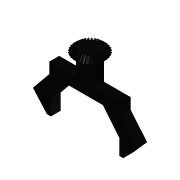
# Autodesk Inventor part: Gripper_Gear
Saved by Autodesk Inventor 2016 (Build 200138000, 138)
## iProperties
Created: 2015-05-21
Part Number: Gripper_Gear
Material: PC/ABS Plastic
Document SubType Name: Modeling
Designer: CHUNGBK
Categories: <?xml version="1.0" encoding="UTF-16"?> <MemberInstance><Categories><FamilyTemplate><FamilyTemplateParameter ValueType="xs:double" Id="1" ObjectReferenceKey="da_z" ObjectType="kUserParameterObject"/><FamilyTemplateParameter ValueType="xs:double" Id="2" ObjectReferenceKey="da_b" ObjectType="kUserParameterObject"/><FamilyTemplateParameter ValueType="xs:double" Id="3" ObjectReferenceKey="da_beta" ObjectType="kUserParameterObject"/><FamilyTemplateParameter ValueType="xs:double" Id="4" ObjectReferenceKey="da_dae" ObjectType="kUserParameterObject"/><FamilyTemplateParameter ValueType="xs:double" Id="5" ObjectReferenceKey="da_ve" ObjectType="kUserParameterObject"/><FamilyTemplateParameter ValueType="xs:double" Id="6" ObjectReferenceKey="da_omega" ObjectType="kUserParameterObject"/><FamilyTemplateParameter ValueType="xs:string" Id="7" ObjectReferenceKey="EAIAABAAAAAAHwAAAAAAAIAAAAAAAAAA" ObjectType="83914240" SubObjectId="SurfaceGeometry"/></FamilyTemplate><ParamToTemplateMap><ParamToTemplate CategoryParameter="//CategoryParameter[@InternalName='046C89C9-8512-4d59-83FE-43B91F4F132A']" TemplateParameter="1"/><ParamToTemplate CategoryParameter="//CategoryParameter[@InternalName='2552DF32-E462-4b46-AEBF-C6C7768E72AC']" TemplateParameter="2"/><ParamToTemplate CategoryParameter="//CategoryParameter[@InternalName='C9EE641D-15FC-4fae-A226-E94C4372FDD7']" TemplateParameter="3"/><ParamToTemplate><ParamToTemplate CategoryParameter="//CategoryParameter[@InternalName='00B6519A-459B-49c7-AD84-2E56D39A5744']" ConstantValue="0.000000"/></ParamToTemplate><ParamToTemplate><ParamToTemplate CategoryParameter="//CategoryParameter[@InternalName='04B31F0E-C7A6-4894-AA32-9629BEFACF47']" ConstantValue="1.000000"/></ParamToTemplate><ParamToTemplate><ParamToTemplate CategoryParameter="//CategoryParameter[@InternalName='43CBEC2E-7847-49e7-A936-2F7889FCB2D9']" ConstantValue="0.200000"/></ParamToTemplate><ParamToTemplate><ParamToTemplate CategoryParameter="//CategoryParameter[@InternalName='B1EFC894-105D-4ebd-86BF-FA20ED196853']" ConstantValue="0.300000"/></ParamToTemplate><ParamToTemplate><ParamToTemplate CategoryParameter="//CategoryParameter[@InternalName='51175063-3D10-4879-93E8-6246FE8B403D']" ConstantValue="2060110000.000000"/></ParamToTemplate><ParamToTemplate><ParamToTemplate CategoryParameter="//CategoryParameter[@InternalName='A3A52E27-4454-46a9-B0BD-C932399B70AF']" ConstantValue="0.300000"/></ParamToTemplate><ParamToTemplate CategoryParameter="//CategoryParameter[@InternalName='2A200944-5A8C-41ca-B96E-8520D2E510F1']" TemplateParameter="4"/><ParamToTemplate><ParamToTemplate CategoryParameter="//CategoryParameter[@InternalName='1A637F62-92C8-44bc-B81F-10802510B579']" ConstantValue="3.585907"/></ParamToTemplate><ParamToTemplate CategoryParameter="//CategoryParameter[@InternalName='B52DD4BE-6863-48fb-BF58-89EF6F9EC65C']" TemplateParameter="5"/><ParamToTemplate><ParamToTemplate CategoryParameter="//CategoryParameter[@InternalName='3956BFF2-84D2-457d-93C2-9B0613DEBA67']" ConstantValue="1.641185"/></ParamToTemplate><ParamToTemplate CategoryParameter="//CategoryParameter[@InternalName='739CFA02-461B-4bf8-8049-181FCAD8B28F']" TemplateParameter="6"/><ParamToTemplate><ParamToTemplate CategoryParameter="//CategoryParameter[@InternalName='A27E999F-E2CE-4481-8A2A-EBF499C4C3C5']" ConstantValue="0.000000"/></ParamToTemplate><ParamToTemplate><ParamToTemplate CategoryParameter="//CategoryParameter[@InternalName='9E1B4470-B2D3-4ff1-B813-535BB4CDF51A']" ConstantValue="3520790.000000"/></ParamToTemplate><ParamToTemplate><ParamToTemplate CategoryParameter="//CategoryParameter[@InternalName='F8452263-BFF6-458c-9FB1-07C4B99E95CD']" ConstantValue="11389170.000000"/></ParamToTemplate><ParamToTemplate><ParamToTemplate CategoryParameter="//CategoryParameter[@InternalName='3E3BB259-FD49-497f-8171-6EBC954A3479']" ConstantValue="2.000000"/></ParamToTemplate><ParamToTemplate CategoryParameter="//CategoryParameter[@InternalName='27C3BAF2-7550-4e4b-AE2C-0DB134B7D9B7']" TemplateParameter="7"/></ParamToTemplateMap><Category DisplayName="Gear" InternalName="DC85795E-93AB-48d5-8EEE-5A27447B64BD" Mnemonic="Gear"><CategoryParameter DisplayName="z" InternalName="046C89C9-8512-4d59-83FE-43B91F4F132A" Mnemonic="z"/><CategoryParameter DisplayName="b" InternalName="2552DF32-E462-4b46-AEBF-C6C7768E72AC" Mnemonic="b"/><CategoryParameter DisplayName="||b|" InternalName="C9EE641D-15FC-4fae-A226-E94C4372FDD7" Mnemonic="beta"/><CategoryParameter DisplayName="x" InternalName="00B6519A-459B-49c7-AD84-2E56D39A5744" Mnemonic="x"/><CategoryParameter DisplayName="a*" InternalName="04B31F0E-C7A6-4894-AA32-9629BEFACF47" Mnemonic="a"/><CategoryParameter DisplayName="c*" InternalName="43CBEC2E-7847-49e7-A936-2F7889FCB2D9" Mnemonic="c"/><CategoryParameter DisplayName="r|.f|*" InternalName="B1EFC894-105D-4ebd-86BF-FA20ED196853" Mnemonic="rf"/><CategoryParameter DisplayName="E" InternalName="51175063-3D10-4879-93E8-6246FE8B403D" Mnemonic="E"/><CategoryParameter DisplayName="||m|" InternalName="A3A52E27-4454-46a9-B0BD-C932399B70AF" Mnemonic="mi"/><Category DisplayName="BevelGear" InternalName="0C98F69A-0C2B-4791-B2FE-7691BB227E77" Mnemonic="BevelGear"><CategoryParameter DisplayName="d|.ae|" InternalName="2A200944-5A8C-41ca-B96E-8520D2E510F1" Mnemonic="dae"/><CategoryParameter DisplayName="d|.ai|" InternalName="1A637F62-92C8-44bc-B81F-10802510B579" Mnemonic="dai"/><CategoryParameter DisplayName="A|.e|" InternalName="B52DD4BE-6863-48fb-BF58-89EF6F9EC65C" Mnemonic="ve"/><CategoryParameter DisplayName="A|.i|" InternalName="3956BFF2-84D2-457d-93C2-9B0613DEBA67" Mnemonic="vi"/><CategoryParameter DisplayName="||S|" InternalName="739CFA02-461B-4bf8-8049-181FCAD8B28F" Mnemonic="omega"/><CategoryParameter DisplayName="x|.t|" InternalName="A27E999F-E2CE-4481-8A2A-EBF499C4C3C5" Mnemonic="xt"/><CategoryParameter DisplayName="||s||.Flim|" InternalName="9E1B4470-B2D3-4ff1-B813-535BB4CDF51A" Mnemonic="sFlim"/><CategoryParameter DisplayName="||s||.Hlim|" InternalName="F8452263-BFF6-458c-9FB1-07C4B99E95CD" Mnemonic="sHlim"/><CategoryParameter DisplayName="type" InternalName="3E3BB259-FD49-497f-8171-6EBC954A3479" Mnemonic="type"/><CategoryParameter DisplayName="PitchDiameter" InternalName="27C3BAF2-7550-4e4b-AE2C-0DB134B7D9B7" Mnemonic="IDS_PITCHDIAM"/></Category></Category></Categories></MemberInstance>
Mass: 60.9118 g
Surface Area: 34.3074 cm^2
Volume: 7.7496 cm^3
Density: 0.357273 g/cm^3
Appearance: Smooth - Black
CustomPartVersion: 1
Author: CHUNGBK
Autodesk Inventor part; units mm, degrees
ref_plane "XZ Plane" through (0, 0, 0) normal (0, 1, 0) x (-1, 0, 0)
ref_plane "Mesh Plane2" through (0, 0, 0) normal (0.9951847, 0.0980171, 0) x (0, 0, 1)
sketch "Teeth Body Sketch" plane through (0, 0, 0) normal (1, 0, 0) x (0, 1, 0)
  line L0 (0, 0) -> (22.638081, -25.173683) construction
  line L1 (22.638081, -25.173683) -> (24.962383, -22.849382)
  line L2 (24.962383, -22.849382) -> (0, 0) construction
  line L3 (23.905882, -23.905882) -> (0, 0) construction
  line L4 (16.260077, -18.081304) -> (17.929535, -16.411846)
  line L5 (22.638081, -25.173683) -> (16.260077, -18.081304)
  line L6 (24.962383, -22.849382) -> (17.929535, -16.411846)
  line L7 (0, -39.386751) -> (0, 6.564458)
  line L8 (0, -23.905882) -> (24.962383, -23.905882) construction
  dimension "d0" = 47.81176
  dimension "d1" = 45.27616
  dimension "d2" = 49.92477
  dimension "d3" = 9.525
  dimension "d4" = 22.84938
  constraints: 16 end point, 4 point on line, 3 perpendicular, 2 collinear, 1 horizontal alignment, 1 vertical alignment
  measures "d0" diameter of L3.start L7
  measures "d1" diameter of L0.end L7
  measures "d2" diameter of L1.end L7
  measures "d3" distance between parallel lines of L1 L4
  measures "d4" vertical distance of L1.end L0.start
revolve "Teeth Body" add sketch "Teeth Body Sketch" angle 360 about axis through (0, 0, 0) along (0, 0, 1)
ref_plane "Tooth Plane" through (0, 23.905882, -23.905882) normal (0, -0.7071068, 0.7071068) x (1, 0, 0)
sketch "Start Sketch" plane through (0, 23.905882, -23.905882) normal (0, -0.7071068, 0.7071068) x (1, 0, 0)
  line L0 (0, -23.505131) -> (0, 10.644758)
  arc A0 (-0.533967, -2.187388) -> (-2.475681, 2.395688) centre (-12.386496, -4.506093) ccw
  arc A1 (2.475681, 2.395688) -> (0.533967, -2.187388) centre (12.386496, -4.506093) ccw
  line L1 (-0.533967, -2.187388) -> (0.533967, -2.187388)
  arc A2 (2.475681, 2.395688) -> (-2.475681, 2.395688) centre (0, -33.808023) ccw
  dimension "d7" = 12.0772
  dimension "d8" = 12.3865
  dimension "d9" = 29.30193
  dimension "d57" = 36.28826
  dimension "d58" = 31.62063
  constraints: 6 point on circle, 3 centre point, 3 symmetric about line, 2 end point, 1 coincident, 1 perpendicular, 1 other
  measures "d7" radius of A0
  measures "d8" horizontal distance of point (0, -33.808) A0.centre
  measures "d9" vertical distance of point (0, -33.808) A0.centre
  measures "d57" radius of A2
  measures "d58" distance from line of A2.centre L1
sketch "End Sketch" plane through (0, 17.054475, -17.054475) normal (0, -0.7071068, 0.7071068) x (1, 0, 0)
  line L0 (0, -15.358918) -> (0, 6.982715)
  arc A0 (-0.381466, -1.528864) -> (-1.768628, 1.745289) centre (-8.848923, -3.185348) ccw
  arc A1 (1.768628, 1.745289) -> (0.381466, -1.528864) centre (8.848923, -3.185348) ccw
  line L1 (-0.381466, -1.528864) -> (0.381466, -1.528864)
  arc A2 (1.768628, 1.745289) -> (-1.768628, 1.745289) centre (0, -24.11867) ccw
  dimension "d12" = 8.62796
  dimension "d15" = 8.84892
  dimension "d16" = 20.93332
  dimension "d59" = 25.92436
  dimension "d60" = 22.58981
  constraints: 6 point on circle, 3 centre point, 3 symmetric about line, 2 end point, 1 coincident, 1 other
  measures "d12" radius of A0
  measures "d15" horizontal distance of A0.centre point (0, -24.119)
  measures "d16" vertical distance of A0.centre point (0, -24.119)
  measures "d59" radius of A2
  measures "d60" distance from line of A2.centre L1
loft "Loft" cut profiles "Start Sketch", "End Sketch"
pattern_circular "Circular Pattern" count 32 over 360 about axis through (0, 0, 0) along (0, 0, 1) of "Loft"
ref_plane "End Plane" through (0, 17.054475, -17.054475) normal (0, -0.7071068, 0.7071068) x (1, 0, 0)
sketch "Body Sketch" plane through (0, 0, 0) normal (1, 0, 0) x (0, 1, 0)
  line L0 (0, -35.037536) -> (0, -19.530831)
  line L1 (22.638081, -25.173683) -> (16.260077, -18.081304)
  line L2 (16.260077, -18.081304) -> (0, -18.081304)
  line L3 (22.638081, -25.173683) -> (0, -25.173683)
  constraints: 4 end point, 2 perpendicular, 2 point on line
sketch "Body Sketch outline for Fix Body" plane through (0, 0, 0) normal (1, 0, 0) x (0, 1, 0)
  line L0 (0, -25.173683) -> (22.638081, -25.173683)
  line L1 (0, -18.081304) -> (0, -25.173683)
  line L2 (16.260077, -18.081304) -> (0, -18.081304)
  line L3 (22.638081, -25.173683) -> (16.260077, -18.081304)
revolve "Fix Body" add sketch "Body Sketch outline for Fix Body" angle 360 about axis through (0, 0, 0) along (0, 0, 1)
sketch "Sketch6" plane through (0, 0, 0) normal (1, 0, 0) x (0, 1, 0)
  line L0 (23.905882, -23.905882) -> (0, 0)
  line L1 (0, -37.799919) -> (0, 6.299986)
surface revolve "Pitch Diameter" sketch "Sketch6" angle 360 about axis through (0, 0, 0) along (0, 0, 1) shown no curves L0
sketch "Sketch8" plane through (0, 0, 0) normal (0, 1, 0) x (-1, 0, 0)
  line L0 (-9.229524, -25.173683) -> (-8.090488, -25.173683)
  line L1 (0.616442, -25.173683) -> (-0.616442, -25.173683)
  line L2 (-0.616442, -25.173683) -> (-3.810236, -25.173683)
  line L3 (-3.810236, -25.173683) -> (-5.01943, -25.173683)
  line L4 (-5.01943, -25.173683) -> (-8.090488, -25.173683)
  line L5 (-8.090488, -25.173683) -> (-9.229524, -25.173683)
  line L6 (-9.229524, -25.173683) -> (-12.059828, -25.173683)
  line L7 (-12.059828, -25.173683) -> (-13.084933, -25.173683)
  line L8 (-13.084933, -25.173683) -> (-15.565715, -25.173683)
  line L9 (-15.565715, -25.173683) -> (-16.437495, -25.173683)
  line L10 (-16.437495, -25.173683) -> (-18.47342, -25.173683)
  line L11 (-18.47342, -25.173683) -> (-19.158374, -25.173683)
  line L12 (-19.158374, -25.173683) -> (-20.671203, -25.173683)
  line L13 (-20.671203, -25.173683) -> (-21.143007, -25.173683)
  line L14 (-21.143007, -25.173683) -> (-22.074602, -25.173683)
  line L15 (-22.074602, -25.173683) -> (-22.315126, -25.173683)
  line L16 (-22.315126, -25.173683) -> (-22.629687, -25.173683)
  line L17 (-22.629687, -25.173683) -> (-22.629687, -25.173683)
  line L18 (-22.629687, -25.173683) -> (-22.315126, -25.173683)
  line L19 (-22.315126, -25.173683) -> (-22.074602, -25.173683)
  line L20 (-22.074602, -25.173683) -> (-21.143007, -25.173683)
  line L21 (-21.143007, -25.173683) -> (-20.671203, -25.173683)
  line L22 (-20.671203, -25.173683) -> (-19.158374, -25.173683)
  line L23 (-19.158374, -25.173683) -> (-18.47342, -25.173683)
  line L24 (-18.47342, -25.173683) -> (-16.437495, -25.173683)
  line L25 (-16.437495, -25.173683) -> (-15.565715, -25.173683)
  line L26 (-15.565715, -25.173683) -> (-13.084933, -25.173683)
  line L27 (-13.084933, -25.173683) -> (-12.059828, -25.173683)
  line L28 (-12.059828, -25.173683) -> (-9.229524, -25.173683)
  line L29 (-9.229524, -25.173683) -> (-8.090488, -25.173683)
  line L30 (-8.090488, -25.173683) -> (-5.01943, -25.173683)
  line L31 (-5.01943, -25.173683) -> (-3.810236, -25.173683)
  line L32 (-3.810236, -25.173683) -> (-0.616442, -25.173683)
  line L33 (-0.616442, -25.173683) -> (0.616442, -25.173683)
  line L34 (0.616442, -25.173683) -> (3.810236, -25.173683)
  line L35 (3.810236, -25.173683) -> (5.01943, -25.173683)
  line L36 (5.01943, -25.173683) -> (8.090488, -25.173683)
  line L37 (8.090488, -25.173683) -> (9.229524, -25.173683)
  line L38 (9.229524, -25.173683) -> (12.059828, -25.173683)
  line L39 (12.059828, -25.173683) -> (13.084933, -25.173683)
  line L40 (13.084933, -25.173683) -> (15.565715, -25.173683)
  line L41 (15.565715, -25.173683) -> (16.437495, -25.173683)
  line L42 (16.437495, -25.173683) -> (18.47342, -25.173683)
  line L43 (18.47342, -25.173683) -> (19.158374, -25.173683)
  line L44 (19.158374, -25.173683) -> (20.671203, -25.173683)
  line L45 (20.671203, -25.173683) -> (21.143007, -25.173683)
  line L46 (21.143007, -25.173683) -> (22.074602, -25.173683)
  line L47 (22.074602, -25.173683) -> (22.315126, -25.173683)
  line L48 (22.315126, -25.173683) -> (22.629687, -25.173683)
  line L49 (22.629687, -25.173683) -> (22.629687, -25.173683)
  line L50 (22.629687, -25.173683) -> (22.315126, -25.173683)
  line L51 (22.315126, -25.173683) -> (22.074602, -25.173683)
  line L52 (22.074602, -25.173683) -> (21.143007, -25.173683)
  line L53 (21.143007, -25.173683) -> (20.671203, -25.173683)
  line L54 (20.671203, -25.173683) -> (19.158374, -25.173683)
  line L55 (19.158374, -25.173683) -> (18.47342, -25.173683)
  line L56 (18.47342, -25.173683) -> (16.437495, -25.173683)
  line L57 (16.437495, -25.173683) -> (15.565715, -25.173683)
  line L58 (15.565715, -25.173683) -> (13.084933, -25.173683)
  line L59 (13.084933, -25.173683) -> (12.059828, -25.173683)
  line L60 (12.059828, -25.173683) -> (9.229524, -25.173683)
  line L61 (9.229524, -25.173683) -> (8.090488, -25.173683)
  line L62 (8.090488, -25.173683) -> (5.01943, -25.173683)
  line L63 (5.01943, -25.173683) -> (3.810236, -25.173683)
  line L64 (3.810236, -25.173683) -> (0.616442, -25.173683)
  line L65 (0, -25.173683) -> (0, -79.148683)
  line L66 (0, -79.148683) -> (28.575, -79.148683)
  line L67 (28.575, -79.148683) -> (54.71189, -111.093771)
  line L68 (54.71189, -111.093771) -> (54.71189, -136.493771)
  line L69 (54.71189, -136.493771) -> (61.06189, -136.493771)
  line L70 (61.06189, -136.493771) -> (83.427944, -111.093771)
  line L71 (83.427944, -111.093771) -> (57.291055, -79.148683)
  line L72 (57.291055, -79.148683) -> (57.291055, -61.686183)
  line L73 (57.291055, -61.686183) -> (14.2875, -61.686183)
  line L74 (14.2875, -61.686183) -> (14.2875, -25.173683)
  line L75 (14.2875, -25.173683) -> (0, -25.173683)
  line L76 (54.71189, -111.093771) -> (83.427944, -111.093771) construction
  point P0 (0, 0)
  dimension "d90" = 14.2875
  dimension "d91" = 53.975
  dimension "d92" = 17.4625
  dimension "d93" = 22.225
  dimension "d94" = 41.275
  dimension "d95" = 6.35
  dimension "d96" = 25.4
  dimension "d97" = 28.575
  constraints: 24 end point, 4 perpendicular, 3 parallel, 3 point on line, 2 horizontal, 1 midpoint, 1 vertical
  measures "d90" distance between parallel lines of L74 L65
  measures "d91" distance of L65.start L65.end
  measures "d92" distance between parallel lines of L73 L66
  measures "d93" distance between parallel lines of L71 L67
  measures "d94" distance of L66.end L67.end
  measures "d95" distance of L68.end L69.end
  measures "d96" distance of L67.end L68.end
  measures "d97" distance from line of L66.end L65
extrude "Extrusion1" add sketch "Sketch8" along normal mid plane 15.875
mirror "Mirror1" about plane through (0, 0, -25.173683) normal (1, 0, 0) of "Extrusion1"
sketch "Sketch9" plane through (0, 0, -18.081304) normal (0, 0, 1) x (0.9951847, 0.0980171, 0)
  circle A0 centre (0, 0) radius 3.175
  dimension "d100" = 6.35
  constraints: 1 centre point, 1 coincident
  measures "d100" diameter of A0
extrude "Extrusion2" cut sketch "Sketch9" against normal blind 2.54
equation "\"d0\" = da_de"
equation "\"d1\" = da_dfe"
equation "\"d2\" = da_dae"
equation "\"d3\" = da_b"
equation "\"d4\" = da_ve"
equation "\"d7\" = fd_rr"
equation "\"d8\" = fd_x"
equation "\"d9\" = fd_y"
equation "\"d57\" = 0.5 * fd_dva + 0.3 * da_he"
equation "\"d58\" = 0.5 * fd_dva - 1.12 * da_he"
equation "\"da_teethtype\" = 0"
equation "\"da_b\" = 9.525"
equation "\"da_de\" = 47.81176"
equation "\"da_dae\" = 49.92477"
equation "\"da_dfe\" = 45.27616"
equation "\"da_le\" = 33.80802"
equation "\"da_omega\" = 90deg"
equation "\"da_beta\" = 0"
equation "\"da_delta\" = 45deg"
equation "\"da_alpha\" = 20deg"
equation "\"da_he\" = 3.28706"
equation "\"da_ve\" = 22.84938"
equation "\"da_zv\" = 45.254834"
equation "\"fd_loft\" = da_b + 0.05 * da_he"
equation "\"fd_x\" = fd_x1 + fd_x2"
equation "\"fd_y\" = fd_y1 - fd_y2"
equation "\"fd_dd\" = fd_dva - 0.8 * da_he"
equation "\"da_dvw\" = 67.61605"
equation "\"d11\" = fd_loft"
equation "\"da_dm\" = 41.07657"
equation "\"da_x\" = 0"
equation "\"da_m\" = 1.49412"
equation "\"d50\" = da_omega"
equation "\"fd_rr\" = 12.077204"
equation "\"fd_dva\" = 70.604281"
equation "\"fd_x1\" = 1.173242"
equation "\"fd_x2\" = 11.213255"
equation "\"fd_y1\" = 33.787659"
equation "\"fd_y2\" = 4.485729"
body "Solid1"
body "Srf1"
